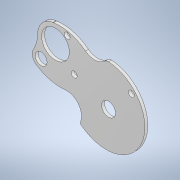
# Autodesk Inventor part: 足内フレーム
Saved by Autodesk Inventor 2022.2 (Build 262287000, 287)
## iProperties
Created: 2022-01-10
Part Number: 足内フレーム
Material: Aluminum 2014-T4
Document SubType Name: Modeling
Designer: acps
Density: 2.8 g/cm^3
Appearance: Satin
Author: acps
Autodesk Inventor part; units mm, degrees
ref_plane "YZ Plane" through (0, 0, 0) normal (1, 0, 0) x (0, 1, 0)
ref_plane "XZ Plane" through (0, 0, 0) normal (0, 1, 0) x (-1, 0, 0)
ref_plane "XY Plane" through (0, 0, 0) normal (0, 0, 1) x (1, 0, 0)
sketch "Sketch2" plane through (0, 0, 0) normal (0, 0, 1) x (1, 0, 0)
  circle A0 centre (46.4683, 30) radius 14
  circle A1 centre (66.4734, 20) radius 20.5 construction
  circle A2 centre (100, 0) radius 30 construction
  circle A3 centre (123.045, 25) radius 3
  circle A4 centre (100, 0) radius 3 construction
  circle A5 centre (32, 10) radius 6.025
  circle A6 centre (32, 10) radius 9
  arc A7 (24.2619, 14.5959) -> (28.4683, 29.9683) centre (-1.5316, 29.9155) ccw
  arc A8 (44, 47.83) -> (28.4683, 29.9683) centre (46.4683, 30) ccw
  arc A9 (110.6259, 39.2116) -> (45.1112, 47.9488) centre (57.174, -111.5959) ccw construction
  arc A10 (91.0837, -36) -> (110.6259, 39.2116) centre (97.597, 2.4523) ccw
  arc A11 (28.683, 27.2278) -> (91.0837, -36) centre (103.7763, 38.9326) ccw construction
  circle A12 centre (58.3063, 43.4) radius 3
  arc A13 (44.5539, 47.9057) -> (44, 47.83) centre (65.9403, -110.6586) ccw
  arc A14 (76.7854, 39.1678) -> (44.5539, 47.9057) centre (50.3015, 5.2915) ccw
  arc A15 (76.7854, 39.1678) -> (96.2775, 40.0369) centre (86.0239, 50.9851) ccw
  arc A16 (100.004, 41.3779) -> (96.2775, 40.0369) centre (99.6954, 36.3875) ccw
  arc A17 (91.0837, -36) -> (100.004, 41.3779) centre (97.597, 2.4523) ccw
  arc A18 (71.7021, -25.434) -> (56.1699, -4.9398) centre (57.7789, -19.8532) ccw
  arc A19 (26.8231, 2.638) -> (56.1699, -4.9398) centre (51.5573, 37.8121) ccw
  arc A20 (71.7021, -25.434) -> (72.3316, -27.7575) centre (73.5586, -26.1781) ccw
  arc A21 (72.3316, -27.7575) -> (91.0837, -36) centre (98.098, 5.4101) ccw
  circle A22 centre (58.3063, 43.4) radius 3
  circle A23 centre (123.045, 25) radius 3
  circle A24 centre (100, 0) radius 3 construction
  circle A25 centre (100, 0) radius 7.025
  circle A26 centre (65.359, 13) radius 3
  point P0 (0, 0)
  point P1 (0, 0)
  point P2 (86.6921, 36)
  point P3 (61.5525, 46.7935)
  point P4 (110.6259, 39.2116)
  dimension "d0" = 12.05
  dimension "d1" = 18
  dimension "d2" = 10
  dimension "d3" = 32
  dimension "d4" = 4
  dimension "d5" = 30
  dimension "d6" = 15
  dimension "d7" = 15
  dimension "d8" = 2
  dimension "d9" = 43
  dimension "d10" = 5
  dimension "d11" = 43
  dimension "d12" = 36
  dimension "d13" = 44
  dimension "d14" = 42
  dimension "d15" = 74
  dimension "d16" = 118
  dimension "d18" = 110.6259
  dimension "d21" = 14.05
  dimension "d22" = 6
  dimension "d23" = 37
  dimension "d24" = 13
  constraints: 31 point on circle, 26 centre point, 14 tangent, 5 coincident, 4 concentric, 17 other
  measures "d0" diameter of A5
  measures "d1" diameter of A6
  measures "d2" vertical distance of point (0, 0) A5.centre
  measures "d3" horizontal distance of point (0, 0) A5.centre
  measures "d4" radial gap between concentric circles of A8 A0
  measures "d5" radius of A7
  measures "d6" radius of A15
  measures "d7" radius of A18
  measures "d8" radius of A20
  measures "d9" radius of A19
  measures "d10" radius of A16
  measures "d11" radius of A14
  measures "d12" vertical distance of point (0, 0) point (86.692, 36)
  measures "d13" horizontal distance of point (0, 0) A8.start
  measures "d14" radius of A21
  measures "d18" horizontal distance of point (0, 0) A10.end
  measures "d21" diameter of A25
  measures "d22" diameter of A26
  measures "d23" distance of A2.centre A26.centre
  measures "d24" vertical distance of point (0, 0) A26.centre
extrude "Extrusion1" add sketch "Sketch2" against normal blind 3
body "Solid1"
